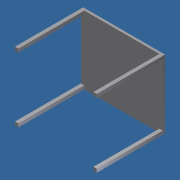
# Autodesk Inventor part: table
Saved by Autodesk Inventor 2012 (Build 160160000, 160)
## iProperties
Created: 2012-11-01
Part Number: table
Material: Default
Document SubType Name: Modeling
Designer: Ed
Density: 1 g/cm^3
Author: Ed
Autodesk Inventor part; units mm, degrees
ref_plane "YZ Plane" through (0, 0, 0) normal (1, 0, 0) x (0, 1, 0)
ref_plane "XZ Plane" through (0, 0, 0) normal (0, 1, 0) x (-1, 0, 0)
ref_plane "XY Plane" through (0, 0, 0) normal (0, 0, 1) x (1, 0, 0)
sketch "Sketch1" plane through (0, 0, 0) normal (0, 0, 1) x (1, 0, 0)
  line L0 (0, 0) -> (914.4, 0)
  line L1 (914.4, 0) -> (914.4, 762)
  line L2 (914.4, 762) -> (0, 762)
  line L3 (0, 762) -> (0, 0)
  dimension "d0" = 914.4
  dimension "d1" = 762
  constraints: 8 end point, 2 parallel, 1 coincident, 1 horizontal, 1 perpendicular
  measures "d0" distance of L0.start L0.end
  measures "d1" distance of L2.end L0.start
extrude "Extrusion1" add sketch "Sketch1" along normal blind 25.4
sketch "Sketch2" plane through (0, 0, 25.4) normal (0, 0, 1) x (1, 0, 0)
  line L0 (0, 762) -> (38.1, 762)
  line L1 (38.1, 762) -> (38.1, 723.9)
  line L2 (38.1, 723.9) -> (0, 723.9)
  line L3 (0, 723.9) -> (0, 762)
  line L4 (914.4, 762) -> (876.3, 762)
  line L5 (876.3, 762) -> (876.3, 723.9)
  line L6 (876.3, 723.9) -> (914.4, 723.9)
  line L7 (914.4, 723.9) -> (914.4, 762)
  line L8 (914.4, 0) -> (876.3, 0)
  line L9 (876.3, 0) -> (876.3, 38.1)
  line L10 (876.3, 38.1) -> (914.4, 38.1)
  line L11 (914.4, 38.1) -> (914.4, 0)
  line L12 (0, 0) -> (38.1, 0)
  line L13 (38.1, 0) -> (38.1, 38.1)
  line L14 (38.1, 38.1) -> (0, 38.1)
  line L15 (0, 38.1) -> (0, 0)
  dimension "d4" = 38.1
  constraints: 32 end point, 8 parallel, 7 perpendicular, 4 collinear, 4 horizontal
  measures "d4" distance of L1.end L2.end
extrude "Extrusion2" add sketch "Sketch2" along normal blind 736.6
body "Solid1"
